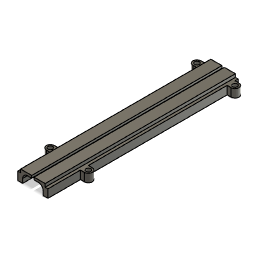
Board Adapter v8 (Autodesk Fusion 360 design; units mm, degrees)
Autodesk Fusion 360 part; units mm, degrees
note: some values were not read from the file. Set by a fixed rule: which sketch regions a step uses.
sketch "Sketch1" plane through (0, 0, 0) normal (0, 0, 1) x (1, 0, 0)
  line L0 (8.75, 5.69) -> (6, 5.69)
  line L1 (3.0466, 2.7352) -> (3.0398, -0.0147)
  line L2 (8.75, 5.69) -> (8.75, 7.19)
  line L3 (8.75, 7.19) -> (1.75, 7.1899)
  line L4 (3.0398, -0.0147) -> (-0.0002, -0.0072)
  line L5 (1.75, 7.1899) -> (1.75, 5.1899)
  line L6 (1.75, 5.1899) -> (0, 5.1899)
  line L7 (0, 5.1899) -> (-0.0002, -0.0072)
  arc A0 (6, 5.69) -> (3.0466, 2.7352) centre (6, 2.7366) ccw
  dimension "d11" = 2.75
  dimension "d12" = 2.75
  dimension "d13" = 1.5
  dimension "d35" = 7
  dimension "d38" = 3.04
  dimension "d39" = 2
  dimension "d40" = 1.75
  dimension "d41" = 5.1971
  constraint horizontal L0
  constraint perpendicular L0 L2
  constraint perpendicular L1 L4
  constraint vertical L5
  constraint perpendicular L5 L6
  constraint tangent L0 A0
  measures "d11" distance of L0.start L0.end
  measures "d12" distance of L1.start L1.end
  measures "d13" distance of L0.start L2.end
  measures "d35" distance of L2.end L3.end
  measures "d38" distance of L1.end L4.end
  measures "d39" distance of L3.end L5.end
  measures "d40" distance of L5.end L6.end
  measures "d41" vertical distance of L4.end L6.end
extrude "Extrude1" add sketch "Sketch1" along normal blind 120 makes body 1
sketch "Sketch2" plane through (0, 5.1899, 0) normal (0, 1, 0) x (-1, 0, 0)
  line L0 (-1.75, 0) -> (0, 0)
  line L1 (0, 0) -> (0, 120)
  line L2 (0, 120) -> (-1.75, 120)
  line L3 (-1.75, 120) -> (-1.75, 0)
  line L4 (0, 0) -> (0, 4.5) construction
  line L5 (0, 4.5) -> (2.5, 4.5) construction
  circle A0 centre (2.5, 4.5) radius 2.5
  line L6 (0, 0) -> (0, 2) construction
  line L7 (0, 2) -> (2.5, 2)
  line L8 (0, 0) -> (0, 7) construction
  line L9 (0, 7) -> (2.5, 7)
  circle A1 centre (2.5, 4.5) radius 1.5
  line L10 (0, 0) -> (0, 97) construction
  line L11 (0, 97) -> (2.5, 97) construction
  circle A2 centre (2.5, 97) radius 2.5
  line L12 (0, 97) -> (0, 94.5)
  line L13 (0, 97) -> (0, 99.5) construction
  line L14 (0, 94.5) -> (2.5, 94.5)
  line L15 (0, 99.5) -> (2.5, 99.5)
  circle A3 centre (2.5, 97) radius 1.5
  line L16 (-1.75, 0) -> (0, 0)
  line L17 (0, 0) -> (0, 120)
  line L18 (0, 120) -> (-1.75, 120)
  line L19 (-1.75, 120) -> (-1.75, 0)
  dimension "d20" = 4.5
  dimension "d21" = 2.5
  dimension "d22" = 5
  dimension "d23" = 2
  dimension "d24" = 7
  dimension "d25" = 3
  dimension "d26" = 97
  dimension "d27" = 2.5
  dimension "d28" = 5
  dimension "d29" = 2.5
  dimension "d30" = 2.5
  dimension "d31" = 3
  constraint vertical L4
  constraint coincident L0.end L1.start
  constraint perpendicular L4 L5
  constraint coincident L5.end A0.centre
  constraint perpendicular L5 L6
  constraint coincident A0 L7.end
  constraint tangent A0 L7
  constraint vertical L8
  constraint coincident A0 L9.end
  constraint tangent A0 L9
  constraint concentric A0 A1
  constraint vertical L10
  constraint perpendicular L10 L11
  constraint coincident L11.end A2.centre
  constraint perpendicular L11 L12
  constraint vertical L13
  constraint coincident A2 L14.end
  constraint tangent A2 L14
  constraint coincident A2 L15.end
  constraint tangent A2 L15
  constraint concentric A2 A3
  measures "d20" distance of L0.end L4.end
  measures "d21" distance of L4.end L5.end
  measures "d22" diameter of A0
  measures "d23" distance of L0.end L6.end
  measures "d24" distance of L0.end L8.end
  measures "d25" diameter of A1
  measures "d26" distance of L0.end L10.end
  measures "d27" distance of L10.end L11.end
  measures "d28" diameter of A2
  measures "d29" distance of L10.end L12.end
  measures "d30" distance of L10.end L13.end
  measures "d31" diameter of A3
extrude "Extrude2" add sketch "Sketch2" against normal blind 5.1971 contours L1 A0 L7 L17 | L1 A0 L9 L17 | A0 | L1 A2 L15 L17 | L1 A2 L12 L14 L17 | A2 bodies 1
mirror "Mirror2" about plane through (0, 0, 0) normal (0, 1, 0) of bodies 1 makes body 2
move_body "Move3" bodies 1 to x (1, 0, 0) y (0, 1, 0) z (0, 0, 1) at (20, 0, 0)
move_body "Move4" bodies 2 to x (-1, 0, 0) y (0, -1, 0) z (0, 0, 1) at (41.9997, -0.1814, 0)
move_body "Move5" bodies 1 to x (1, 0, 0) y (0, 1, 0) z (0, 0, 1) at (-20, 0, 0)
move_body "Move6" bodies 2 to x (1, 0, 0) y (0, 1, 0) z (0, 0, 1) at (-23, 0, 0)
sketch "Sketch3" plane through (0, -0.0071, 0) normal (-0.002166, -0.999998, 0) x (0, 0, 1)
  line L0 (0, 0.0001) -> (0, -3.5399)
  line L1 (0, -3.5399) -> (120, -3.5399)
  line L2 (120, -3.5399) -> (120, 0.0001)
  line L3 (120, 0.0001) -> (99.5, 0.0001)
  line L4 (99.5, 0.0001) -> (94.5, 0.0001)
  line L5 (94.5, 0.0001) -> (7, 0.0001)
  line L6 (7, 0.0001) -> (2, 0.0001)
  line L7 (2, 0.0001) -> (0, 0.0001)
equation "d23 = 4.5 mm - 2.5 mm"
equation "d24 = 4.5 mm + 2.5 mm"
named bodies: "Right", "Left"
